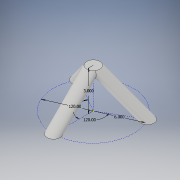
# Autodesk Inventor part: CameraTripodBase
Saved by Autodesk Inventor 2018.1 (Build 221171000, 171)
## iProperties
Created: 2017-10-28
Part Number: CameraTripodBase
Material: Generic
Document SubType Name: Modeling
Designer: steele
Density: 1 g/cm^3
Appearance: Default
Author: steele
Autodesk Inventor part; units mm, degrees
ref_plane "YZ Plane" through (0, 0, 0) normal (1, 0, 0) x (0, 1, 0)
ref_plane "XY Plane" through (0, 0, 0) normal (0, 0, 1) x (1, 0, 0)
sketch "Sketch1" plane through (0, 0, 0) normal (0, 1, 0) x (-1, 0, 0)
  circle A0 centre (0, 0) radius 76.2 construction
  line L0 (0, 0) -> (0, 76.2) construction
  line L1 (0, 0) -> (65.9911, -38.1) construction
  line L2 (0, 0) -> (-65.9911, -38.1) construction
  dimension "d0" = 152.4
  dimension "d1" = 120
  dimension "d2" = 120
  constraints: 6 end point, 3 point on circle, 1 centre point, 1 coincident, 1 vertical
  measures "d0" diameter of A0
  measures "d1" angle of L1 L0
  measures "d2" angle of L2 L0
sketch "Sketch2" plane through (0, 0, 0) normal (1, 0, 0) x (0, 1, 0)
  line L0 (0, 0) -> (76.2, 0) construction
  dimension "d3" = 76.2
  constraints: 2 end point, 1 horizontal
  measures "d3" distance of L0.start L0.end
ref_plane "Work Plane1" through (0, 76.2, 0) normal (0, 1, 0) x (-1, 0, 0)
sketch "Sketch3" plane through (0, 76.2, 0) normal (0, 1, 0) x (-1, 0, 0)
  circle A0 centre (0, 0) radius 12.7
  dimension "d5" = 25.4
  constraints: 1 centre point, 1 coincident
  measures "d5" diameter of A0
sketch3d "3D Sketch1"
  line L0 (0, 76.2, 0) -> (0, 0, 76.2)
sweep "Sweep2" add profiles "Sketch3" path "3D Sketch1"
sketch "Sketch4" plane through (0, 76.2, 0) normal (0, 1, 0) x (-1, 0, 0)
  circle A0 centre (0, 0) radius 12.7
  constraints: 1 centre point, 1 coincident
sketch3d "3D Sketch2"
  line L0 (0, 76.2, 0) -> (65.9911, 0, -38.1)
sweep "Sweep3" add profiles "Sketch4" path "3D Sketch2"
sketch "Sketch5" plane through (0, 76.2, 0) normal (0, 1, 0) x (-1, 0, 0)
  circle A0 centre (0, 0) radius 12.7
  constraints: 1 centre point, 1 coincident
sketch3d "3D Sketch3"
  line L0 (0, 76.2, 0) -> (-65.9911, 0, -38.1)
sweep "Sweep4" add profiles "Sketch5" path "3D Sketch3"
body "Solid2"
